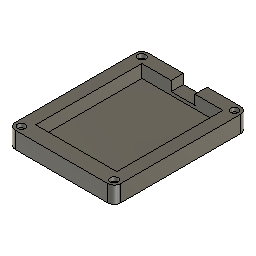
Macropad_Case (Autodesk Fusion 360 design; units mm, degrees)
Autodesk Fusion 360 part; units mm, degrees
sketch "Sketch1" plane through (0, 0, 0) normal (0, 0, 1) x (1, 0, 0)
  line L0 (-22.0435, 48.4594) -> (40.8695, 48.4594)
  line L1 (40.8695, 48.4594) -> (40.8695, -33.8746)
  line L2 (40.8695, -33.8746) -> (-22.0435, -33.8746)
  line L3 (-22.0435, -33.8746) -> (-22.0435, 48.4594)
  line L4 (-31.5435, 57.9594) -> (50.3695, 57.9594)
  line L5 (50.3695, 57.9594) -> (50.3695, -45.3846)
  line L6 (50.3695, -45.3846) -> (-31.5435, -45.3846)
  line L7 (-31.5435, -45.3846) -> (-31.5435, 57.9594)
  circle A0 centre (-26.5435, -40.3846) radius 1.7
  circle A1 centre (45.3695, -40.3846) radius 1.7
  circle A2 centre (45.3695, 52.9594) radius 1.7
  circle A3 centre (-26.5435, 52.9594) radius 1.7
  circle A4 centre (-26.5435, -40.3846) radius 3
  circle A5 centre (45.3695, -40.3846) radius 3
  circle A6 centre (45.3695, 52.9594) radius 3
  circle A7 centre (-26.5435, 52.9594) radius 3
  line L8 (25, 50) -> (-15, 50) construction
  line L9 (-15, 50) -> (-15, 55) construction
  line L10 (-15, 55) -> (25, 55) construction
  line L11 (25, 55) -> (25, 50) construction
  dimension "d1" = 62.913
  dimension "d2" = 82.334
  dimension "d3" = 81.913
  dimension "d4" = 103.344
  dimension "d5" = 9.5
  dimension "d6" = 9.5
  dimension "d7" = 3.4
  dimension "d8" = 5
  dimension "d9" = 5
  dimension "d10" = 3.4
  dimension "d11" = 5
  dimension "d12" = 5
  dimension "d13" = 3.4
  dimension "d14" = 5
  dimension "d15" = 5
  dimension "d16" = 3.4
  dimension "d17" = 5
  dimension "d18" = 5
  dimension "d19" = 6
  dimension "d20" = 6
  dimension "d21" = 6
  dimension "d22" = 6
  dimension "d43" = 2
  text T0 "Matts Universal Macropad" font "Arial" height 2 align left top in box 40 x 5 at (25, 50) x (-1, 0) y (0, 1) spacing 1
  constraint horizontal L0
  constraint vertical L1
  constraint horizontal L2
  constraint vertical L3
  constraint horizontal L4
  constraint vertical L5
  constraint horizontal L6
  constraint vertical L7
  constraint concentric A0 A4
  constraint concentric A1 A5
  constraint concentric A2 A6
  constraint concentric A3 A7
  measures "d1" distance of L0.start L0.end
  measures "d2" distance of L0.start L2.end
  measures "d3" distance of L4.start L4.end
  measures "d4" distance of L4.start L6.end
  measures "d5" distance of L0 L4
  measures "d6" distance of L3 L7
  measures "d7" diameter of A0
  measures "d8" distance of L7 A0.centre
  measures "d9" distance of L6 A0.centre
  measures "d10" diameter of A1
  measures "d11" distance of L5 A1.centre
  measures "d12" distance of L6 A1.centre
  measures "d13" diameter of A2
  measures "d14" distance of L4 A2.centre
  measures "d15" distance of L5 A2.centre
  measures "d16" diameter of A3
  measures "d17" distance of L4 A3.centre
  measures "d18" distance of L7 A3.centre
  measures "d19" diameter of A4
  measures "d20" diameter of A5
  measures "d21" diameter of A6
  measures "d22" diameter of A7
extrude "Extrude1" add sketch "Sketch1" along normal blind 9.9 contours A4 | A5 | A6 | A7 makes body 1 at (42.3732, 52.8098, 6.6) makes body 2 at (-23.5473, 52.8098, 6.6) makes body 3 at (42.3732, -40.5342, 6.6) makes body 4 at (-29.5398, -40.5342, 6.6)
extrude "Extrude2" add sketch "Sketch1" along normal blind 13 contours L4 L5 L6 L7 bodies 1 2 3 4
extrude "Extrude3" add sketch "Sketch1" along normal blind 3 contours L0 L1 L2 L3 bodies 1
sketch "Sketch2" plane through (0, 0, 13) normal (0, 0, 1) x (-1, 0, 0)
  circle A0 centre (26.5435, 40.3846) radius 3
  circle A1 centre (-45.3695, -52.9594) radius 3
  circle A2 centre (-45.3695, 40.3846) radius 3
  circle A3 centre (26.5435, -52.9594) radius 3
  line L0 (-40.8695, 33.8746) -> (22.0435, 33.8746)
  line L1 (22.0435, 33.8746) -> (22.0435, -48.4594)
  line L2 (22.0435, -48.4594) -> (-40.8695, -48.4594)
  line L3 (-40.8695, -48.4594) -> (-40.8695, 33.8746)
  line L4 (31.5435, 45.3846) -> (-50.3695, 45.3846)
  line L5 (-50.3695, 45.3846) -> (-50.3695, -57.9594)
  line L6 (-50.3695, -57.9594) -> (31.5435, -57.9594)
  line L7 (31.5435, -57.9594) -> (31.5435, 45.3846)
  line L8 (-19.1675, -57.9594) -> (-0.6675, -57.9594)
  line L9 (-0.6675, -57.9594) -> (-0.6675, -48.4594)
  line L10 (-0.6675, -48.4594) -> (-19.1675, -48.4594)
  line L11 (-19.1675, -48.4594) -> (-19.1675, -57.9594)
  line L12 (31.5435, 45.3846) -> (31.5435, -57.9594)
  dimension "d29" = 32.211
  dimension "d30" = 18.5
  constraint horizontal L8
  constraint vertical L9
  constraint horizontal L10
  constraint vertical L11
  constraint coincident L2 L9.end
  constraint coincident L6 L8.start
  measures "d29" distance of L9 L12
  measures "d30" distance of L9 L11
fillet "Fillet4" radius 5 4 edges at (-31.5435, -45.3846, 6.5) (50.3695, -45.3846, 6.5) (50.3695, 57.9594, 6.5) (-31.5435, 57.9594, 6.5) on bodies 1
extrude "Extrude5" cut sketch "Sketch2" against normal blind 7.5 contours L2 L6 L8 L9 L10 L11 bodies 1
extrude "Extrude6" cut sketch "Sketch1" along normal blind 2 text T0 bodies 1
extrude "Extrude4" [suppressed]
fillet "Fillet1" [suppressed]
fillet "Fillet2" [suppressed]
fillet "Fillet3" [suppressed]
equation "d44 = 'Matts Universal Macropad'"
